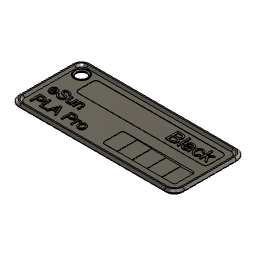
filament_sample (Autodesk Fusion 360 design; units mm, degrees)
Autodesk Fusion 360 part; units mm, degrees
sketch "base_sketch" plane through (0, 0, 0) normal (0, 0, 1) x (1, 0, 0)
  line L0 (5, 0) -> (75, 0)
  line L1 (80, -5) -> (80, -30)
  line L2 (75, -35) -> (5, -35)
  line L3 (0, -30) -> (0, -5)
  line L4 (13.5, -5) -> (73.5, -5)
  line L5 (75, -6.5) -> (75, -13.5)
  line L6 (73.5, -15) -> (13.5, -15)
  line L7 (5, -15) -> (5, -5)
  line L8 (68, -20) -> (75, -20)
  line L9 (75, -20) -> (75, -30)
  line L10 (75, -30) -> (68, -30)
  line L11 (68, -30) -> (68, -20)
  line L12 (68, -30) -> (61, -30)
  line L13 (61, -30) -> (61, -20)
  line L14 (61, -20) -> (68, -20)
  line L15 (68, -20) -> (68, -30)
  line L16 (61, -30) -> (54, -30)
  line L17 (54, -30) -> (54, -20)
  line L18 (54, -20) -> (61, -20)
  line L19 (61, -20) -> (61, -30)
  line L20 (54, -30) -> (47, -30)
  line L21 (47, -30) -> (47, -20)
  line L22 (47, -20) -> (54, -20)
  line L23 (54, -20) -> (54, -30)
  line L24 (47, -30) -> (40, -30)
  line L25 (40, -30) -> (40, -20)
  line L26 (40, -20) -> (47, -20)
  line L27 (47, -20) -> (47, -30)
  circle A0 centre (6.5, -6.5) radius 2.5
  line L28 (12, -6.5) -> (12, -13.5)
  line L29 (5, -17) -> (38, -17)
  line L30 (38, -17) -> (38, -30)
  line L31 (38, -30) -> (5, -30)
  line L32 (5, -30) -> (5, -17)
  arc A1 (5, 0) -> (0, -5) centre (5, -5) ccw
  arc A2 (80, -5) -> (75, 0) centre (75, -5) ccw
  arc A3 (75, -35) -> (80, -30) centre (75, -30) ccw
  arc A4 (0, -30) -> (5, -35) centre (5, -30) ccw
  line L33 (75, -32.4) -> (5, -32.4)
  arc A5 (2.6, -30) -> (5, -32.4) centre (5, -30) ccw
  line L34 (2.6, -30) -> (2.6, -5)
  arc A6 (5, -2.6) -> (2.6, -5) centre (5, -5) ccw
  line L35 (5, -2.6) -> (75, -2.6)
  arc A7 (77.4, -5) -> (75, -2.6) centre (75, -5) ccw
  line L36 (77.4, -5) -> (77.4, -30)
  arc A8 (75, -32.4) -> (77.4, -30) centre (75, -30) ccw
  arc A9 (13.5, -5) -> (12, -6.5) centre (13.5, -6.5) ccw
  arc A10 (12, -13.5) -> (13.5, -15) centre (13.5, -13.5) ccw
  arc A11 (75, -6.5) -> (73.5, -5) centre (73.5, -6.5) ccw
  arc A12 (73.5, -15) -> (75, -13.5) centre (73.5, -13.5) ccw
  line L37 (5, -23.5) -> (38, -23.5) construction
  line L38 (38, -23.5) -> (38, -17) construction
  line L39 (38, -17) -> (5, -17) construction
  line L40 (5, -17) -> (5, -23.5) construction
  line L41 (5, -30) -> (38, -30) construction
  line L42 (38, -30) -> (38, -23.5) construction
  line L43 (38, -23.5) -> (5, -23.5) construction
  line L44 (5, -23.5) -> (5, -30) construction
  line L45 (13.5, -15) -> (73.5, -15) construction
  line L46 (73.5, -15) -> (73.5, -5) construction
  line L47 (73.5, -5) -> (13.5, -5) construction
  line L48 (13.5, -5) -> (13.5, -15) construction
  circle A13 centre (6.5, -6.5) radius 3.5
  point P0 (80, 0)
  point P1 (0, -35)
  point P2 (75, -5)
  point P3 (75, -15)
  dimension "d1" = 80
  dimension "d2" = 35
  dimension "d22" = 10
  dimension "d23" = 5
  dimension "d24" = 5
  dimension "d25" = 5
  dimension "d32" = 5
  dimension "d33" = 5
  dimension "d34" = 10
  dimension "d35" = 7
  dimension "d38" = -28
  dimension "d39" = 0
  dimension "d43" = 5
  dimension "d44" = 2.6
  dimension "d46" = 7
  dimension "d52" = 2
  dimension "d55" = 2
  dimension "d58" = 5
  dimension "d59" = 1.5
  dimension "d78" = 5
  dimension "d79" = 5
  dimension "d86" = 6
  dimension "d87" = 6.5
  dimension "d88" = 6.5
  dimension "d91" = 1
  text T0 "eSun" font "Arial" height 5 align left top in box 33 x 6.5 at (5, -23.5) x (1, 0) y (0, 1) spacing 1
  text T1 "PLA Pro" font "Arial" height 5 align left bottom in box 33 x 6.5 at (5, -30) x (1, 0) y (0, 1) spacing 1
  text T2 "Black" font "Arial" height 6 align right middle in box 60 x 10 at (13.5, -15) x (1, 0) y (0, 1) spacing 1
  constraint horizontal L0
  constraint vertical L1
  constraint horizontal L2
  constraint vertical L3
  constraint horizontal L4
  constraint vertical L5
  constraint horizontal L6
  constraint vertical L7
  constraint horizontal L8
  constraint vertical L9
  constraint horizontal L10
  constraint vertical L11
  constraint perpendicular L6 L28
  constraint horizontal L29
  constraint vertical L30
  constraint horizontal L31
  constraint vertical L32
  constraint collinear L7 L32
  constraint collinear L10 L31
  constraint coincident origin L0
  constraint coincident origin L3
  constraint tangent L0 A1
  constraint tangent L3 A1
  constraint coincident P0 L0
  constraint coincident P0 L1
  constraint tangent L0 A2
  constraint tangent L1 A2
  constraint equal A1 A2
  constraint tangent L1 A3
  constraint tangent L2 A3
  constraint equal A1 A3
  constraint coincident P1 L2
  constraint coincident P1 L3
  constraint tangent L2 A4
  constraint tangent L3 A4
  constraint equal A1 A4
  constraint coincident L7.end L4
  constraint tangent L4 A9
  constraint tangent L28 A9
  constraint coincident L7.start L6
  constraint tangent L28 A10
  constraint tangent L6 A10
  constraint equal A9 A10
  constraint coincident P2 L4
  constraint coincident P2 L5
  constraint tangent L4 A11
  constraint tangent L5 A11
  constraint equal A9 A11
  constraint coincident P3 L5
  constraint coincident P3 L6
  constraint tangent L5 A12
  constraint tangent L6 A12
  constraint equal A9 A12
  constraint midpoint L30
  constraint coincident L29.start
  constraint coincident L30.end
  constraint coincident L6.start
  constraint coincident L4.start
  measures "d1" distance of origin P0
  measures "d2" distance of origin P1
  measures "d22" distance of P2 P3
  measures "d23" distance of L0 L4
  measures "d24" distance of L1 L5
  measures "d25" distance of L3 L7
  measures "d32" distance of L1 L9
  measures "d33" distance of L2 L10
  measures "d34" distance of L8.start L10.end
  measures "d35" distance of L9.end L10.end
  measures "d43" diameter of A0
  measures "d46" distance of L7 L28
  measures "d52" distance of L25 L30
  measures "d55" distance of L6 L29
  measures "d58" radius of A1
  measures "d59" radius of A9
  measures "d87" distance of L0 A0.centre
  measures "d88" distance of L3 A0.centre
extrude "ext_12" add sketch "base_sketch" along normal blind 1.2 contours L29 L30 L31 L32 | L33 A5 L34 A6 L35 A7 L36 A8
extrude "ext_22" add sketch "base_sketch" along normal blind 2.2 contours L0 L1 L2 L3 A1 A2 A3 A4
extrude "ext_14" add sketch "base_sketch" along normal blind 1.4 contours A13
extrude "ext_10" add sketch "base_sketch" along normal blind 1 contours L4 L5 L6 L28 A9 A10 A11 A12 | L21 L24 L25 L26 L27
extrude "ext_08" add sketch "base_sketch" along normal blind 0.8 contours L17 L20 L21 L22 L23 L27
extrude "ext_06" add sketch "base_sketch" along normal blind 0.6 contours L13 L16 L17 L18 L19 L23
extrude "ext_04" add sketch "base_sketch" along normal blind 0.4 contours L11 L12 L13 L14 L15 L19
extrude "ext_02" add sketch "base_sketch" along normal blind 0.2 contours L8 L9 L10 L11 L15
fillet "fillet_pattern_edges" radius 1 4 edges at (40, -20, 1.1) (75, -30, 0.7) (75, -20, 0.7) (40, -30, 1.1)
chamfer "chamfer_body_sides" distance 1 angle 45 24 edges at (40, -35, 2.2) (78.5355, -33.5355, 2.2) (80, -17.5, 2.2) (78.5355, -1.4645, 2.2) (40, 0, 2.2) (1.4645, -1.4645, 2.2) (0, -17.5, 2.2) (1.4645, -33.5355, 2.2) (40, -32.4, 2.2) (3.3029, -31.6971, 2.2) (2.6, -17.5, 2.2) (3.3029, -3.3029, 2.2) (40, -2.6, 2.2) (76.6971, -3.3029, 2.2) (77.4, -17.5, 2.2) (76.6971, -31.6971, 2.2) (40, -35, 0) (1.4645, -33.5355, 0) (0, -17.5, 0) (1.4645, -1.4645, 0) (40, 0, 0) (78.5355, -1.4645, 0) (80, -17.5, 0) (78.5355, -33.5355, 0)
extrude "extrude_color" add sketch "base_sketch" along normal blind 1.4 text T2
extrude "extrude_brand_and_type" add sketch "base_sketch" along normal blind 1.6 text T0 T1
chamfer "chamfer_ring_hole" distance 0.2 angle 45 1 edges at (3.2369, -7.7657, 1.4)
fillet "fillet_ring_hole" radius 0.5 2 edges at (4.1692, -5.596, 1.4) (4.1692, -5.596, 0)
named bodies: "filament_sample"
